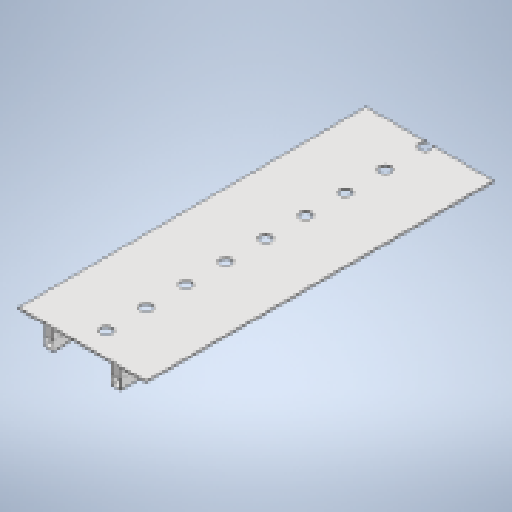
# Autodesk Inventor part: ДМФ 067 крышка v2.0
Saved by Autodesk Inventor 2026.2 (Build 302298000, 298)
## iProperties
Created: 2024-06-28
Part Number: ДМФ 067 крышка v2.0
Material: Generic
Document SubType Name: Sheet Metal
Designer: admin
Density: 1 g/cm^3
Sheet Metal Rule: Default
Appearance: Default
Author: admin
Autodesk Inventor part; units mm, degrees
ref_plane "YZ Plane" through (0, 0, 0) normal (1, 0, 0) x (0, 1, 0)
ref_plane "XZ Plane" through (0, 0, 0) normal (0, 1, 0) x (-1, 0, 0)
ref_plane "XY Plane" through (0, 0, 0) normal (0, 0, 1) x (1, 0, 0)
sketch "Sketch1" plane through (0, 0, 0) normal (0, 0, 1) x (1, 0, 0)
  line L0 (-400, -1080) -> (400, -1080)
  line L1 (400, -1080) -> (400, 1080)
  line L2 (400, 1080) -> (-400, 1080)
  line L3 (-400, 1080) -> (-400, -1080)
  line L4 (-400, -1080) -> (400, 1080) construction
  line L5 (400, -1080) -> (-400, 1080) construction
  point P0 (0, 0)
  dimension "d0" = 800
  dimension "d1" = 2160
  measures "d0" distance of L2.end L1.end
  measures "d1" distance of L1.end L0.end
extrude "Plate1" add sketch "Sketch1" along normal blind 10
sketch "Sketch2" plane through (0, 0, 10) normal (0, 0, 1) x (1, 0, 0)
  line L0 (400, -1080) -> (-400, -1080) projected
  line L1 (400, 1080) -> (400, -1080) projected
  line L2 (-400, 1080) -> (400, 1080) projected
  line L3 (-400, -1080) -> (-400, 1080) projected
  circle A0 centre (0, -929.5) radius 35
  point P0 (0, 0)
  point P1 (0, -1080)
  dimension "d3" = 70
  dimension "d4" = 150.5
  constraints: 1 centre point, 1 midpoint, 1 vertical alignment
  measures "d3" diameter of A0
  measures "d4" distance from line of L0 A0.centre
extrude "Extrusion1" cut sketch "Sketch2" against normal through all contours A0
pattern_linear "Rectangular Pattern1" count 9 spacing 250 along (0, 1, 0) of "Extrusion1"
sketch "Sketch3" plane through (0, 0, 0) normal (0, 0, -1) x (-1, 0, 0)
  line L0 (240, -1080) -> (180, -1080)
  line L1 (180, -1080) -> (180, 1080)
  line L2 (180, 1080) -> (240, 1080)
  line L3 (240, 1080) -> (240, -1080)
  line L4 (-180, -1080) -> (-240, -1080)
  line L5 (-240, -1080) -> (-240, 1080)
  line L6 (-240, 1080) -> (-180, 1080)
  line L7 (-180, 1080) -> (-180, -1080)
  line L8 (0, -1080) -> (0, 1305.1217) construction
  line L9 (400, -1080) -> (-400, -1080) projected
  line L10 (-400, 1080) -> (400, 1080) projected
  point P0 (0, 0)
  dimension "d10" = 60
  dimension "d11" = 360
  constraints: 18 end point, 5 collinear, 4 parallel, 2 horizontal, 2 perpendicular, 1 midpoint, 1 vertical, 1 other
  measures "d10" distance between parallel lines of L1 L3
  measures "d11" distance between parallel lines of L7 L1
extrude "Extrusion2" add sketch "Sketch3" along normal blind 60 contours L0 L1 L2 L3 | L4 L5 L6 L7
sketch "Sketch4" plane through (-400, 1080, 10) normal (0, 1, 0) x (1, 0, 0)
  line L0 (160, 70) -> (220, 70) projected
  line L1 (160, 70) -> (220, 70)
  line L2 (220, 70) -> (220, 130)
  line L3 (220, 130) -> (160, 130)
  line L4 (160, 130) -> (160, 70)
  line L5 (163, 127) -> (217, 127)
  line L6 (217, 127) -> (217, 73)
  line L7 (217, 73) -> (163, 73)
  line L8 (163, 73) -> (163, 127)
  point P0 (400, 10)
  dimension "d15" = 60
  dimension "d16" = 3
  constraints: 16 end point, 4 parallel, 2 perpendicular, 1 horizontal, 3 other
  measures "d15" distance of L3.end L0.start
  measures "d16" distance between parallel lines of L3 L5
extrude "Extrusion3" add sketch "Sketch4" against normal up to surface (2160 mm away)
mirror "Mirror1" about plane through (0, 0, 0) normal (1, 0, 0) of "Extrusion3"
equation "\"d2\" = Thickness"
equation "\"BendReliefDepth\" = 0.5 * Thickness"
equation "\"Thickness\" = 10"
body "Solid1"
